Autodesk Fusion 360 part; units mm, degrees
(part 2 of 2)
sketch "Sketch5" plane through (0, 0, 14.5) normal (0, 0, 1) x (-1, 0, 0)
  line L0 (7.35, 0.35) -> (-89.35, 0.35)
  line L1 (-89.35, 0.35) -> (-89.35, -86.85)
  line L2 (-89.35, -86.85) -> (7.35, -86.85)
  line L3 (7.35, -86.85) -> (7.35, 0.35)
  spline S0 degree 3 poles (-37.3382, -76.3676) (-37.0226, -76.1422) (-36.3689, -75.6012) (-35.8504, -75.1052) knots 0 0 0 0 1 1 1 1
  line L4 (-35.8504, -75.1052) -> (-34.9262, -74.2261)
  line L5 (-34.9262, -74.2261) -> (-33.1455, -74.6093)
  spline S1 degree 3 poles (-33.1455, -74.6093) (-30.6659, -75.1278) (-28.1638, -74.97) (-26.4732, -74.2036) knots 0 0 0 0 1 1 1 1
  spline S2 degree 3 poles (-26.4732, -74.2036) (-23.385, -72.7835) (-21.5817, -69.6277) (-21.5592, -65.5928) knots 0 0 0 0 1 1 1 1
  spline S3 degree 3 poles (-21.5592, -65.5928) (-21.5366, -64.646) (-21.4014, -64.2177) (-20.6575, -63.1132) knots 0 0 0 0 1 1 1 1
  spline S4 degree 3 poles (-20.6575, -63.1132) (-19.7333, -61.7156) (-19.3726, -60.3406) (-19.6206, -59.1234) knots 0 0 0 0 1 1 1 1
  spline S5 degree 3 poles (-19.6206, -59.1234) (-19.7784, -58.2442) (-20.4321, -56.8918) (-20.6575, -56.8918) knots 0 0 0 0 1 1 1 1
  spline S6 degree 3 poles (-20.6575, -56.8918) (-20.7702, -56.8918) (-22.1002, -58.2217) (-23.633, -59.8672) knots 0 0 0 0 1 1 1 1
  spline S7 degree 3 poles (-23.633, -59.8672) (-25.1658, -61.4902) (-27.5101, -63.9923) (-28.84, -65.4124) knots 0 0 0 0 1 1 1 1
  spline S8 degree 3 poles (-28.84, -65.4124) (-30.1925, -66.8325) (-31.8381, -68.726) (-32.4918, -69.6277) knots 0 0 0 0 1 1 1 1
  spline S9 degree 3 poles (-32.4918, -69.6277) (-33.8442, -71.4535) (-35.3771, -72.8736) (-36.6168, -73.4823) knots 0 0 0 0 1 1 1 1
  spline S10 degree 3 poles (-36.6168, -73.4823) (-37.9693, -74.136) (-39.9755, -74.1134) (-46.1293, -73.3696) knots 0 0 0 0 1 1 1 1
  spline S11 degree 3 poles (-46.1293, -73.3696) (-49.2851, -72.9863) (-52.3958, -72.6031) (-53.0045, -72.5355) knots 0 0 0 0 1 1 1 1
  line L6 (-53.0045, -72.5355) -> (-54.1315, -72.4228)
  line L7 (-54.1315, -72.4228) -> (-55.3037, -74.181)
  spline S12 degree 3 poles (-55.3037, -74.181) (-56.3181, -75.6913) (-56.4308, -75.9618) (-56.0926, -76.0745) knots 0 0 0 0 1 1 1 1
  spline S13 degree 3 poles (-56.0926, -76.0745) (-55.5517, -76.2774) (-45.3178, -76.7282) (-41.2604, -76.7282) knots 0 0 0 0 1 1 1 1
  spline S14 degree 3 poles (-41.2604, -76.7282) (-38.5103, -76.7282) (-37.789, -76.6606) (-37.3382, -76.3676) knots 0 0 0 0 1 1 1 1
  spline S15 degree 3 poles (-62.1338, -75.3081) (-60.0825, -74.6995) (-57.9185, -73.4146) (-56.8591, -72.1974) knots 0 0 0 0 1 1 1 1
  spline S16 degree 3 poles (-56.8591, -72.1974) (-55.8221, -70.9576) (-54.5598, -68.5231) (-54.1315, -66.9002) knots 0 0 0 0 1 1 1 1
  spline S17 degree 3 poles (-54.1315, -66.9002) (-53.7483, -65.435) (-53.7033, -62.482) (-54.0414, -60.9492) knots 0 0 0 0 1 1 1 1
  spline S18 degree 3 poles (-54.0414, -60.9492) (-54.4697, -58.9881) (-54.5147, -58.2442) (-54.2893, -57.9737) knots 0 0 0 0 1 1 1 1
  spline S19 degree 3 poles (-54.2893, -57.9737) (-54.1766, -57.816) (-53.9512, -57.32) (-53.8385, -56.8918) knots 0 0 0 0 1 1 1 1
  spline S20 degree 3 poles (-53.8385, -56.8918) (-53.7033, -56.4635) (-52.5762, -53.1048) (-51.3139, -49.4531) knots 0 0 0 0 1 1 1 1
  spline S21 degree 3 poles (-51.3139, -49.4531) (-48.8794, -42.3976) (-48.5413, -41.3156) (-48.654, -41.248) knots 0 0 0 0 1 1 1 1
  spline S22 degree 3 poles (-48.654, -41.248) (-49.8937, -40.3463) (-54.0865, -38.6107) (-57.1972, -37.709) knots 0 0 0 0 1 1 1 1
  spline S23 degree 3 poles (-57.1972, -37.709) (-59.8796, -36.9426) (-63.1481, -36.2889) (-63.5313, -36.4467) knots 0 0 0 0 1 1 1 1
  spline S24 degree 3 poles (-63.5313, -36.4467) (-63.8244, -36.5594) (-64.2752, -37.7766) (-65.7404, -42.6907) knots 0 0 0 0 1 1 1 1
  spline S25 degree 3 poles (-65.7404, -42.6907) (-66.1236, -43.9981) (-66.5293, -45.3055) (-66.642, -45.621) knots 0 0 0 0 1 1 1 1
  spline S26 degree 3 poles (-66.642, -45.621) (-66.7547, -45.9366) (-67.0929, -47.1088) (-67.431, -48.2133) knots 0 0 0 0 1 1 1 1
  spline S27 degree 3 poles (-67.431, -48.2133) (-67.7691, -49.3404) (-68.2876, -51.031) (-68.6031, -52.0228) knots 0 0 0 0 1 1 1 1
  spline S28 degree 3 poles (-68.6031, -52.0228) (-68.8962, -52.9921) (-69.0991, -53.8261) (-69.054, -53.8937) knots 0 0 0 0 1 1 1 1
  spline S29 degree 3 poles (-69.054, -53.8937) (-68.9863, -53.9388) (-68.0396, -53.8712) (-66.9125, -53.7134) knots 0 0 0 0 1 1 1 1
  line L8 (-66.9125, -53.7134) -> (-64.8838, -53.4655)
  line L9 (-64.8838, -53.4655) -> (-63.058, -47.8526)
  spline S30 degree 3 poles (-63.058, -47.8526) (-62.0436, -44.787) (-61.1419, -42.2173) (-61.0518, -42.1497) knots 0 0 0 0 1 1 1 1
  spline S31 degree 3 poles (-61.0518, -42.1497) (-60.8263, -42.0144) (-54.943, -43.9304) (-54.65, -44.2235) knots 0 0 0 0 1 1 1 1
  spline S32 degree 3 poles (-54.65, -44.2235) (-54.4922, -44.3813) (-55.1684, -46.7256) (-56.4758, -50.6478) knots 0 0 0 0 1 1 1 1
  line L10 (-56.4758, -50.6478) -> (-58.5271, -56.8467)
  line L11 (-58.5271, -56.8467) -> (-57.9636, -57.816)
  spline S33 degree 3 poles (-57.9636, -57.816) (-56.5886, -60.2279) (-56.1152, -63.6317) (-56.8365, -66.0436) knots 0 0 0 0 1 1 1 1
  spline S34 degree 3 poles (-56.8365, -66.0436) (-57.6255, -68.7035) (-60.4206, -71.3634) (-63.3059, -72.2425) knots 0 0 0 0 1 1 1 1
  spline S35 degree 3 poles (-63.3059, -72.2425) (-64.9965, -72.7609) (-67.4535, -72.7609) (-69.1667, -72.2425) knots 0 0 0 0 1 1 1 1
  spline S36 degree 3 poles (-69.1667, -72.2425) (-71.4208, -71.5437) (-73.8328, -69.1994) (-74.8246, -66.7424) knots 0 0 0 0 1 1 1 1
  spline S37 degree 3 poles (-74.8246, -66.7424) (-75.4332, -65.2546) (-75.4783, -61.8058) (-74.8922, -60.2955) knots 0 0 0 0 1 1 1 1
  spline S38 degree 3 poles (-74.8922, -60.2955) (-74.3287, -58.7852) (-74.4188, -58.3795) (-75.3205, -57.9512) knots 0 0 0 0 1 1 1 1
  spline S39 degree 3 poles (-75.3205, -57.9512) (-75.7713, -57.7483) (-76.1545, -57.568) (-76.1996, -57.568) knots 0 0 0 0 1 1 1 1
  spline S40 degree 3 poles (-76.1996, -57.568) (-76.2447, -57.568) (-76.5828, -58.2442) (-76.9209, -59.1008) knots 0 0 0 0 1 1 1 1
  spline S41 degree 3 poles (-76.9209, -59.1008) (-77.5296, -60.4984) (-77.5746, -60.814) (-77.5521, -63.4288) knots 0 0 0 0 1 1 1 1
  spline S42 degree 3 poles (-77.5521, -63.4288) (-77.5296, -65.8407) (-77.4394, -66.4719) (-76.9886, -67.7117) knots 0 0 0 0 1 1 1 1
  spline S43 degree 3 poles (-76.9886, -67.7117) (-74.6893, -73.8429) (-68.2876, -77.1114) (-62.1338, -75.3081) knots 0 0 0 0 1 1 1 1
  spline S44 degree 3 poles (-38.037, -71.9494) (-36.8648, -71.6339) (-35.3996, -70.5293) (-34.6557, -69.4248) knots 0 0 0 0 1 1 1 1
  spline S45 degree 3 poles (-34.6557, -69.4248) (-32.2213, -65.8858) (-33.957, -60.7463) (-38.1497, -59.1459) knots 0 0 0 0 1 1 1 1
  spline S46 degree 3 poles (-38.1497, -59.1459) (-39.4571, -58.65) (-39.6149, -58.65) (-45.656, -58.7852) knots 0 0 0 0 1 1 1 1
  spline S47 degree 3 poles (-45.656, -58.7852) (-49.0597, -58.8529) (-51.945, -59.0107) (-52.0577, -59.1234) knots 0 0 0 0 1 1 1 1
  spline S48 degree 3 poles (-52.0577, -59.1234) (-52.1704, -59.2361) (-52.1479, -60.025) (-51.9676, -61.0394) knots 0 0 0 0 1 1 1 1
  spline S49 degree 3 poles (-51.9676, -61.0394) (-51.6069, -63.3837) (-51.8323, -66.2014) (-52.5762, -68.5457) knots 0 0 0 0 1 1 1 1
  spline S50 degree 3 poles (-52.5762, -68.5457) (-52.9143, -69.5826) (-53.1397, -70.4617) (-53.0946, -70.5068) knots 0 0 0 0 1 1 1 1
  spline S51 degree 3 poles (-53.0946, -70.5068) (-52.9368, -70.6646) (-40.4263, -72.2199) (-39.5923, -72.1974) knots 0 0 0 0 1 1 1 1
  spline S52 degree 3 poles (-39.5923, -72.1974) (-39.164, -72.1974) (-38.4652, -72.0847) (-38.037, -71.9494) knots 0 0 0 0 1 1 1 1
  spline S53 degree 3 poles (-64.2526, -70.6646) (-62.0887, -70.1461) (-60.105, -68.5682) (-59.023, -66.4719) knots 0 0 0 0 1 1 1 1
  spline S54 degree 3 poles (-59.023, -66.4719) (-58.482, -65.48) (-58.4144, -65.0968) (-58.4144, -63.0907) knots 0 0 0 0 1 1 1 1
  spline S55 degree 3 poles (-58.4144, -63.0907) (-58.4144, -61.0619) (-58.482, -60.7238) (-59.0456, -59.6418) knots 0 0 0 0 1 1 1 1
  spline S56 degree 3 poles (-59.0456, -59.6418) (-61.0292, -55.8774) (-65.4473, -54.3897) (-69.2343, -56.2155) knots 0 0 0 0 1 1 1 1
  spline S57 degree 3 poles (-69.2343, -56.2155) (-70.5643, -56.8692) (-72.1422, -58.4922) (-72.886, -60.0025) knots 0 0 0 0 1 1 1 1
  spline S58 degree 3 poles (-72.886, -60.0025) (-73.427, -61.1296) (-73.5172, -61.5578) (-73.5172, -63.3161) knots 0 0 0 0 1 1 1 1
  spline S59 degree 3 poles (-73.5172, -63.3161) (-73.5172, -65.1194) (-73.4496, -65.5026) (-72.8409, -66.6522) knots 0 0 0 0 1 1 1 1
  spline S60 degree 3 poles (-72.8409, -66.6522) (-71.263, -69.7855) (-67.6339, -71.4535) (-64.2526, -70.6646) knots 0 0 0 0 1 1 1 1
  spline S61 degree 3 poles (-30.1249, -64.2403) (-29.4487, -63.4513) (-27.7355, -61.4902) (-26.3154, -59.9123) knots 0 0 0 0 1 1 1 1
  spline S62 degree 3 poles (-26.3154, -59.9123) (-22.9793, -56.1254) (-22.3932, -55.3364) (-22.7088, -54.9532) knots 0 0 0 0 1 1 1 1
  spline S63 degree 3 poles (-22.7088, -54.9532) (-23.0244, -54.57) (-26.5634, -53.195) (-31.0266, -51.7072) knots 0 0 0 0 1 1 1 1
  spline S64 degree 3 poles (-31.0266, -51.7072) (-35.2869, -50.2871) (-37.0677, -50.0617) (-38.5103, -50.783) knots 0 0 0 0 1 1 1 1
  spline S65 degree 3 poles (-38.5103, -50.783) (-40.494, -51.7298) (-42.2297, -53.9839) (-42.6129, -56.0803) knots 0 0 0 0 1 1 1 1
  line L12 (-42.6129, -56.0803) -> (-42.7707, -56.9594)
  line L13 (-42.7707, -56.9594) -> (-41.4858, -56.8241)
  spline S66 degree 3 poles (-41.4858, -56.8241) (-38.8935, -56.5536) (-36.3463, -57.4778) (-34.3852, -59.3939) knots 0 0 0 0 1 1 1 1
  spline S67 degree 3 poles (-34.3852, -59.3939) (-33.1004, -60.6562) (-31.9733, -62.8652) (-31.7704, -64.5784) knots 0 0 0 0 1 1 1 1
  spline S68 degree 3 poles (-31.7704, -64.5784) (-31.7028, -65.187) (-31.5676, -65.6829) (-31.4999, -65.6604) knots 0 0 0 0 1 1 1 1
  spline S69 degree 3 poles (-31.4999, -65.6604) (-31.4323, -65.6604) (-30.8011, -65.0067) (-30.1249, -64.2403) knots 0 0 0 0 1 1 1 1
  spline S70 degree 3 poles (-59.812, -55.1561) (-59.4739, -54.5925) (-56.7013, -45.7563) (-56.7689, -45.4632) knots 0 0 0 0 1 1 1 1
  spline S71 degree 3 poles (-56.7689, -45.4632) (-56.8365, -45.1026) (-59.7669, -44.0882) (-60.0149, -44.3362) knots 0 0 0 0 1 1 1 1
  spline S72 degree 3 poles (-60.0149, -44.3362) (-60.1501, -44.4714) (-62.5846, -52.113) (-62.9002, -53.3528) knots 0 0 0 0 1 1 1 1
  spline S73 degree 3 poles (-62.9002, -53.3528) (-63.0129, -53.8712) (-62.9678, -54.0065) (-62.4719, -54.1868) knots 0 0 0 0 1 1 1 1
  spline S74 degree 3 poles (-62.4719, -54.1868) (-62.1788, -54.2995) (-61.48, -54.6151) (-60.9616, -54.863) knots 0 0 0 0 1 1 1 1
  spline S75 degree 3 poles (-60.9616, -54.863) (-59.8796, -55.3815) (-59.9472, -55.3589) (-59.812, -55.1561) knots 0 0 0 0 1 1 1 1
  spline S76 degree 3 poles (-21.1534, -52.9921) (-21.0182, -52.8343) (-19.4403, -49.7461) (-17.6369, -46.1395) knots 0 0 0 0 1 1 1 1
  line L14 (-17.6369, -46.1395) -> (-14.3459, -39.5349)
  line L15 (-14.3459, -39.5349) -> (-12.8131, -38.8135)
  spline S77 degree 3 poles (-12.8131, -38.8135) (-10.6942, -37.7766) (-8.395, -35.4549) (-7.2904, -33.2232) knots 0 0 0 0 1 1 1 1
  spline S78 degree 3 poles (-7.2904, -33.2232) (-5.8478, -30.2929) (-5.6674, -26.9567) (-6.7945, -23.7108) knots 0 0 0 0 1 1 1 1
  spline S79 degree 3 poles (-6.7945, -23.7108) (-7.9667, -20.3521) (-10.852, -17.5795) (-14.4811, -16.2946) knots 0 0 0 0 1 1 1 1
  spline S80 degree 3 poles (-14.4811, -16.2946) (-16.1943, -15.7085) (-19.6882, -15.4831) (-21.3563, -15.8663) knots 0 0 0 0 1 1 1 1
  spline S81 degree 3 poles (-21.3563, -15.8663) (-23.6555, -16.3848) (-25.8195, -17.602) (-27.5552, -19.3377) knots 0 0 0 0 1 1 1 1
  spline S82 degree 3 poles (-27.5552, -19.3377) (-30.1024, -21.8849) (-31.0266, -24.1616) (-31.3647, -28.8277) knots 0 0 0 0 1 1 1 1
  spline S83 degree 3 poles (-31.3647, -28.8277) (-31.4774, -30.5634) (-31.9733, -34.711) (-32.4918, -38.4078) knots 0 0 0 0 1 1 1 1
  spline S84 degree 3 poles (-32.4918, -38.4078) (-32.5594, -38.9713) (-32.7623, -40.4365) (-32.92, -41.6763) knots 0 0 0 0 1 1 1 1
  spline S85 degree 3 poles (-32.92, -41.6763) (-33.1004, -42.9161) (-33.3709, -44.8997) (-33.5287, -46.0944) knots 0 0 0 0 1 1 1 1
  spline S86 degree 3 poles (-33.5287, -46.0944) (-33.6865, -47.2666) (-33.7541, -48.3936) (-33.6865, -48.5965) knots 0 0 0 0 1 1 1 1
  spline S87 degree 3 poles (-33.6865, -48.5965) (-33.5963, -48.7994) (-32.5368, -49.2728) (-31.1393, -49.7461) knots 0 0 0 0 1 1 1 1
  line L16 (-31.1393, -49.7461) -> (-28.7499, -50.5576)
  line L17 (-28.7499, -50.5576) -> (-28.4343, -49.8363)
  spline S88 degree 3 poles (-28.4343, -49.8363) (-27.9384, -48.7318) (-25.256, -42.4427) (-24.1063, -39.6476) knots 0 0 0 0 1 1 1 1
  line L18 (-24.1063, -39.6476) -> (-23.0694, -37.1905)
  line L19 (-23.0694, -37.1905) -> (-23.6104, -36.8299)
  spline S89 degree 3 poles (-23.6104, -36.8299) (-27.8031, -34.0798) (-29.5388, -30.4732) (-28.795, -26.1227) knots 0 0 0 0 1 1 1 1
  spline S90 degree 3 poles (-28.795, -26.1227) (-28.0962, -22.1103) (-24.8727, -18.7742) (-20.928, -17.9176) knots 0 0 0 0 1 1 1 1
  spline S91 degree 3 poles (-20.928, -17.9176) (-15.0221, -16.6778) (-9.1614, -20.6451) (-8.2597, -26.5284) knots 0 0 0 0 1 1 1 1
  spline S92 degree 3 poles (-8.2597, -26.5284) (-7.5158, -31.3974) (-10.604, -36.1762) (-15.473, -37.5963) knots 0 0 0 0 1 1 1 1
  spline S93 degree 3 poles (-15.473, -37.5963) (-16.3295, -37.8668) (-17.4115, -37.957) (-18.9669, -37.9344) knots 0 0 0 0 1 1 1 1
  line L20 (-18.9669, -37.9344) -> (-21.221, -37.8668)
  line L21 (-21.221, -37.8668) -> (-21.9424, -39.332)
  spline S94 degree 3 poles (-21.9424, -39.332) (-22.7989, -41.0451) (-26.9691, -50.6929) (-26.9691, -50.9859) knots 0 0 0 0 1 1 1 1
  spline S95 degree 3 poles (-26.9691, -50.9859) (-26.9691, -51.0761) (-26.2252, -51.4367) (-25.3461, -51.7523) knots 0 0 0 0 1 1 1 1
  spline S96 degree 3 poles (-25.3461, -51.7523) (-24.4445, -52.0679) (-23.1821, -52.5413) (-22.5284, -52.7892) knots 0 0 0 0 1 1 1 1
  spline S97 degree 3 poles (-22.5284, -52.7892) (-21.6493, -53.1499) (-21.3112, -53.195) (-21.1534, -52.9921) knots 0 0 0 0 1 1 1 1
  spline S98 degree 3 poles (-48.0454, -38.5881) (-47.6171, -37.4385) (-47.2564, -35.9282) (-47.2564, -35.2971) knots 0 0 0 0 1 1 1 1
  spline S99 degree 3 poles (-47.2564, -35.2971) (-47.2564, -34.0573) (-48.2482, -32.3892) (-49.3528, -31.8482) knots 0 0 0 0 1 1 1 1
  spline S100 degree 3 poles (-49.3528, -31.8482) (-49.8712, -31.5777) (-50.322, -31.3298) (-50.3671, -31.3072) knots 0 0 0 0 1 1 1 1
  spline S101 degree 3 poles (-50.3671, -31.3072) (-50.3897, -31.2847) (-50.2319, -30.7211) (-49.9614, -30.09) knots 0 0 0 0 1 1 1 1
  spline S102 degree 3 poles (-49.9614, -30.09) (-49.2175, -28.1965) (-49.2626, -28.1514) (-51.3815, -27.4977) knots 0 0 0 0 1 1 1 1
  spline S103 degree 3 poles (-51.3815, -27.4977) (-54.3119, -26.5961) (-54.2668, -26.5961) (-54.8529, -28.0387) knots 0 0 0 0 1 1 1 1
  line L22 (-54.8529, -28.0387) -> (-55.3488, -29.2785)
  line L23 (-55.3488, -29.2785) -> (-56.5886, -29.2109)
  spline S104 degree 3 poles (-56.5886, -29.2109) (-58.2566, -29.1207) (-59.564, -29.7068) (-60.6686, -31.0367) knots 0 0 0 0 1 1 1 1
  spline S105 degree 3 poles (-60.6686, -31.0367) (-61.3899, -31.8933) (-62.3592, -33.8093) (-62.3592, -34.3729) knots 0 0 0 0 1 1 1 1
  spline S106 degree 3 poles (-62.3592, -34.3729) (-62.3592, -34.463) (-61.6829, -34.6434) (-60.8489, -34.8011) knots 0 0 0 0 1 1 1 1
  spline S107 degree 3 poles (-60.8489, -34.8011) (-58.8878, -35.1393) (-53.3426, -36.8524) (-50.6151, -37.9795) knots 0 0 0 0 1 1 1 1
  spline S108 degree 3 poles (-50.6151, -37.9795) (-48.2031, -38.9713) (-48.1806, -38.9713) (-48.0454, -38.5881) knots 0 0 0 0 1 1 1 1
  spline S109 degree 3 poles (-16.1492, -35.8155) (-12.4073, -34.7786) (-9.7474, -30.9015) (-10.1757, -27.092) knots 0 0 0 0 1 1 1 1
  spline S110 degree 3 poles (-10.1757, -27.092) (-10.3786, -25.3112) (-11.5958, -22.8993) (-12.8356, -21.8173) knots 0 0 0 0 1 1 1 1
  spline S111 degree 3 poles (-12.8356, -21.8173) (-15.3603, -19.6082) (-19.2825, -18.9996) (-22.2805, -20.3295) knots 0 0 0 0 1 1 1 1
  spline S112 degree 3 poles (-22.2805, -20.3295) (-27.3748, -22.5611) (-28.5695, -29.6166) (-24.5572, -33.629) knots 0 0 0 0 1 1 1 1
  spline S113 degree 3 poles (-24.5572, -33.629) (-22.3707, -35.8155) (-19.1698, -36.6495) (-16.1492, -35.8155) knots 0 0 0 0 1 1 1 1
  spline S114 degree 3 poles (-33.4385, -25.4014) (-33.3709, -25.2887) (-33.2582, -24.8604) (-33.168, -24.4321) knots 0 0 0 0 1 1 1 1
  spline S115 degree 3 poles (-33.168, -24.4321) (-32.875, -22.9894) (-31.2971, -20.0365) (-30.0798, -18.6615) knots 0 0 0 0 1 1 1 1
  spline S116 degree 3 poles (-30.0798, -18.6615) (-24.8051, -12.6655) (-16.3746, -11.6962) (-9.6122, -16.2946) knots 0 0 0 0 1 1 1 1
  line L24 (-9.6122, -16.2946) -> (-8.3273, -17.1737)
  line L25 (-8.3273, -17.1737) -> (-8.1695, -16.0241)
  spline S117 degree 3 poles (-8.1695, -16.0241) (-8.1019, -15.3704) (-8.0343, -13.5671) (-8.0343, -11.9892) knots 0 0 0 0 1 1 1 1
  line L26 (-8.0343, -11.9892) -> (-8.0343, -9.1039)
  line L27 (-8.0343, -9.1039) -> (-22.3481, -9.1039)
  line L28 (-22.3481, -9.1039) -> (-36.6619, -9.1039)
  line L29 (-36.6619, -9.1039) -> (-36.6619, -17.3315)
  line L30 (-36.6619, -17.3315) -> (-36.6619, -25.5592)
  line L31 (-36.6619, -25.5592) -> (-35.1066, -25.5592)
  spline S118 degree 3 poles (-35.1066, -25.5592) (-34.2274, -25.5592) (-33.4836, -25.4915) (-33.4385, -25.4014) knots 0 0 0 0 1 1 1 1
  line L32 (-40.1893, -6.8228) -> (-89.35, -6.8228) construction
  line L33 (-89.35, -6.8228) -> (-89.35, -25.5592) construction
  line L34 (-89.35, -25.5592) -> (-40.1893, -25.5592) construction
  line L35 (-40.1893, -25.5592) -> (-40.1893, -6.8228) construction
  dimension "d134" = 5
  text T0 "J&M AUTOMATION" font "Arial" height 5 align centre middle in box 49.1607 x 18.7363 at (-40.1893, -6.8228) x (-1, 0) y (0, -1) spacing 1
  constraint coincident L1
extrude "Extrude4'" cut sketch "Sketch5" sketch "Sketch5" against normal blind 0.2 contours S0 L4 L5 S1 S2 S3 S4 S5 S6 S7 S8 S9 S10 S11 L6 L7 S12 S13 S14 | S15 S16 S17 S18 S19 S20 S21 S22 S23 S24 S25 S26 S27 S28 S29 L8 L9 S30 S31 S32 L10 L11 S33 S34 S35 S36 S37 S38 S39 S40 S41 S42 S43 | S44 S45 S46 S47 S48 S49 S50 S51 S52 | S53 S54 S55 S56 S57 S58 S59 S60 | S61 S62 S63 S64 S65 L12 L13 S66 S67 S68 S69 | S70 S71 S72 S73 S74 S75 | S76 L14 L15 S77 S78 S79 S80 S81 S82 S83 S84 S85 S86 S87 L16 L17 S88 L18 L19 S89 S90 S91 S92 S93 L20 L21 S94 S95 S96 S97 | S98 S99 S100 S101 S102 S103 L22 L23 S104 S105 S106 S107 S108 | S109 S110 S111 S112 S113 | S114 S115 S116 L24 L25 S117 L26 L27 L28 L29 L30 L31 S118 sketch seen with x (1, 0, 0) y (0, 1, 0) z (0, 0, 1) at (0, 0, 1) of sketch 2 text T0 sketch seen with x (1, 0, 0) y (0, 1, 0) z (0, 0, 1) at (0, 0, 1) bodies 8 in component "kansi"
sketch "Sketch7" plane through (0, 0, 2) normal (0, 0, 1) x (-1, 0, 0)
  circle A0 centre (4.85, -56.85) radius 1.5
  circle A1 centre (-86.85, -56.85) radius 1.5
  circle A2 centre (4.85, -29.65) radius 1.5
  circle A3 centre (-86.85, -29.65) radius 1.5
  line L0 (-47.8333, -32.9988) -> (-47.8333, -31.9988)
  arc A4 (-47.8333, -31.9988) -> (-42.9833, -27.1469) centre (-47.8333, -27.1488) ccw
  line L1 (-42.9833, -27.1469) -> (-41.9833, -27.1465)
  arc A5 (-47.8333, -32.9988) -> (-41.9833, -27.1465) centre (-47.8333, -27.1488) ccw
  line L2 (-4.5, -32.9988) -> (-4.5, -31.9988)
  arc A6 (-4.5, -31.9988) -> (0.35, -27.1469) centre (-4.5, -27.1488) ccw
  line L3 (0.35, -27.1469) -> (1.35, -27.1465)
  arc A7 (-4.5, -32.9988) -> (1.35, -27.1465) centre (-4.5, -27.1488) ccw
  line L4 (2.35, -81.85) -> (-84.35, -81.85)
  line L5 (-84.35, -81.85) -> (-84.35, -79.85)
  line L6 (-84.35, -79.85) -> (2.35, -79.85)
  line L7 (2.35, -79.85) -> (2.35, -81.85)
  line L8 (-61.6835, -27.1499) -> (-60.6832, -27.1499)
  arc A8 (-60.6832, -27.1499) -> (-55.8332, -31.9997) centre (-55.8335, -27.15) ccw
  line L9 (-55.8332, -31.9997) -> (-55.8335, -33)
  arc A9 (-61.6835, -27.1499) -> (-55.8335, -33) centre (-55.8335, -27.15) ccw
  line L10 (-18.3501, -27.1499) -> (-17.3498, -27.1499)
  arc A10 (-17.3498, -27.1499) -> (-12.4999, -31.9997) centre (-12.5001, -27.15) ccw
  line L11 (-12.4999, -31.9997) -> (-12.5002, -33)
  arc A11 (-18.3501, -27.1499) -> (-12.5002, -33) centre (-12.5001, -27.15) ccw
  circle A12 centre (-101.85, -43.25) radius 2.5
  line L12 (-40.0168, -27.1499) -> (-39.0165, -27.1499)
  arc A13 (-39.0165, -27.1499) -> (-34.1666, -31.9997) centre (-34.1668, -27.15) ccw
  line L13 (-34.1666, -31.9997) -> (-34.1668, -33)
  arc A14 (-40.0168, -27.1499) -> (-34.1668, -33) centre (-34.1668, -27.15) ccw
  line L14 (-69.5, -32.9988) -> (-69.5, -31.9988)
  arc A15 (-69.5, -31.9988) -> (-64.65, -27.1469) centre (-69.5, -27.1488) ccw
  line L15 (-64.65, -27.1469) -> (-63.65, -27.1465)
  arc A16 (-69.5, -32.9988) -> (-63.65, -27.1465) centre (-69.5, -27.1488) ccw
  line L16 (-83.3501, -27.1499) -> (-82.3498, -27.1499)
  arc A17 (-82.3498, -27.1499) -> (-77.4999, -31.9997) centre (-77.5001, -27.15) ccw
  line L17 (-77.4999, -31.9997) -> (-77.5002, -33)
  arc A18 (-83.3501, -27.1499) -> (-77.5002, -33) centre (-77.5001, -27.15) ccw
  line L18 (-26.1667, -32.9988) -> (-26.1667, -31.9988)
  arc A19 (-26.1667, -31.9988) -> (-21.3167, -27.1469) centre (-26.1667, -27.1488) ccw
  line L19 (-21.3167, -27.1469) -> (-20.3167, -27.1465)
  arc A20 (-26.1667, -32.9988) -> (-20.3167, -27.1465) centre (-26.1667, -27.1488) ccw
  line L20 (27.35, -22.0462) -> (7.35, -2.0462)
  line L21 (7.35, -2.0462) -> (7.35, 0.35)
  line L22 (7.35, 0.35) -> (2.35, 0.35)
  line L23 (2.35, 0.35) -> (2.35, -9.85)
  line L24 (2.35, -9.85) -> (-84.35, -9.85)
  line L25 (-84.35, -9.85) -> (-84.35, 0.35)
  line L26 (-84.35, 0.35) -> (-89.35, 0.35)
  line L27 (-89.35, 0.35) -> (-89.35, -18.25)
  line L28 (-89.35, -18.25) -> (-109.35, -38.25)
  line L29 (-109.35, -38.25) -> (-109.35, -48.25)
  line L30 (-109.35, -48.25) -> (-89.35, -68.25)
  line L31 (-89.35, -68.25) -> (-89.35, -86.85)
  line L32 (-89.35, -86.85) -> (7.35, -86.85)
  line L33 (7.35, -86.85) -> (7.35, -52.0462)
  line L34 (7.35, -52.0462) -> (27.35, -32.0462)
  line L35 (27.35, -32.0462) -> (27.35, -22.0462)
sketch "Sketch8" plane through (0, -0.35, 0) normal (0, -1, 0) x (1, 0, 0)
  line L0 (17, 12) -> (17, 13)
  line L1 (17, 13) -> (21.6675, 13)
  line L2 (21.6675, 13) -> (21.6675, 12)
  line L3 (21.6675, 12) -> (38.6675, 12)
  line L4 (38.6675, 12) -> (38.6675, 13)
  line L5 (38.6675, 13) -> (43.335, 13)
  line L6 (43.335, 13) -> (43.335, 12)
  line L7 (43.335, 12) -> (60.335, 12)
  line L8 (60.335, 12) -> (60.335, 13)
  line L9 (60.335, 13) -> (65.0025, 13)
  line L10 (65.0025, 13) -> (65.0025, 12)
  line L11 (65.0025, 12) -> (82, 12)
  line L12 (82, 12) -> (82, 13)
  line L13 (82, 13) -> (84.35, 13)
  line L14 (84.35, 13) -> (84.35, 2)
  line L15 (84.35, 2) -> (89.35, 2)
  line L16 (89.35, 2) -> (89.35, 14.5)
  line L17 (89.35, 14.5) -> (-7.35, 14.5)
  line L18 (-7.35, 14.5) -> (-7.35, 2)
  line L19 (-7.35, 2) -> (-2.35, 2)
  line L20 (-2.35, 2) -> (-2.35, 13)
  line L21 (-2.35, 13) -> (0, 13)
  line L22 (0, 13) -> (0, 12)
  line L23 (0, 12) -> (17, 12)
  circle A0 centre (-10.1, 10.25) radius 2.75
  line L24 (-7.35, 13) -> (-7.35, 14.5)
  line L25 (-7.35, 7.6) -> (-7.35, 6)
  line L26 (-7.35, 14.5) -> (-13.35, 14.5)
  line L27 (-7.35, 6) -> (-13.35, 6)
  line L28 (-13.35, 14.5) -> (-13.35, 12.5)
  line L29 (-13.35, 6) -> (-13.35, 8)
  line L30 (-13.35, 8) -> (-11.6811, 8)
  line L31 (-13.35, 12.5) -> (-11.6811, 12.5)
  point P0 (-4.85, 2)
  dimension "d135" = 5.5
  dimension "d136" = 2.75
  dimension "d140" = 6
  dimension "d141" = 6
  dimension "d142" = 2
  dimension "d143" = 2
  dimension "d146" = 4.25
  dimension "d154" = 4.25
  constraint coincident L18 L24.start
  constraint coincident L18 L25.start
  constraint perpendicular L19 L25
  constraint perpendicular L18 L26
  constraint perpendicular L18 L27
  constraint perpendicular L26 L28
  constraint perpendicular L27 L29
  constraint coincident A0 L30.end
  constraint perpendicular L29 L30
  constraint coincident A0 L31.end
  constraint perpendicular L28 L31
  constraint coincident L17.end L18.start
  measures "d135" diameter of A0
  measures "d136" distance of L18 A0.centre
  measures "d140" distance of L17.end L26.end
  measures "d141" distance of L25.end L27.end
  measures "d142" distance of L26.end L28.end
  measures "d143" distance of L27.end L29.end
  measures "d146" distance of L17 A0.centre
  measures "d154" distance of A0.centre L27
extrude "Extrude6'" add sketch "Sketch8" against normal blind 15 contours L18 A0 L25 L27 L29 L30 | L18 A0 L24 L26 L28 L31 sketch seen with x (1, 0, 0) y (0, 1, 0) z (0, 0, 1) at (0, 0, 1) bodies 8 in component "kansi"
sketch "Sketch9" plane through (0, 86.85, 0) normal (0, 1, 0) x (-1, 0, 0)
  line L0 (-89.35, 14.5) -> (-89.35, 2)
  line L1 (-89.35, 2) -> (7.35, 2)
  line L2 (7.35, 2) -> (7.35, 14.5)
  line L3 (7.35, 14.5) -> (-89.35, 14.5)
  line L4 (-49, 2) -> (-33, 2)
  line L5 (-33, 2) -> (-33, 6)
  line L6 (-33, 6) -> (-49, 6)
  line L7 (-49, 6) -> (-49, 2)
  dimension "d147" = 16
  dimension "d148" = 4
  dimension "d149" = 40.35
  constraint horizontal L4
  constraint vertical L5
  constraint horizontal L6
  constraint vertical L7
  constraint coincident L1 L4.start
  measures "d147" distance of L4.start L4.end
  measures "d148" distance of L4.start L6.end
  measures "d149" distance of L0 L7
extrude "Extrude3''" cut sketch "Sketch9" against normal blind 10 contours L1 L4 L5 L6 L7 bodies 7 in component "boksi"
extrude "Extrude7'" cut sketch "Sketch9" against normal blind 10 contours L1 L4 L5 L6 L7 sketch seen with x (1, 0, 0) y (0, 1, 0) z (0, 0, 1) at (0, 0, 1) bodies 8 in component "kansi"
component "boksi" placed x (1, 0, 0) y (0, 1, 0) z (0, 0, 1) at (0, 0, 0)
component "kansi" placed x (1, 0, 0) y (0, 1, 0) z (0, 0, 1) at (0, 0, -1)
equation "d56 = 9 mm + ( 0.35 * 2 ) * 1 mm + 0.5 mm"
equation "d95 = ( 35.3799163327 mm + 41.82 mm ) / 2"
equation "d107 = 1 mm + 1.5 mm"
equation "d110 = 1 mm + 1.5 mm"
equation "d114 = 1 mm + 1.5 mm"
equation "d117 = 1 mm + 1.5 mm"
equation "d118 = 5 mm - 0.6 mm"
equation "d119 = 5 mm - 0.6 mm"
equation "d120 = 5 mm - 0.6 mm"
equation "d121 = 5 mm - 0.6 mm"
equation "d122 = -2 mm - 6 mm"
equation "d124 = -2 mm - 6 mm"
equation "d136 = ( 5.5 / 2 ) * 1 mm"
equation "d141 = 5.5 mm + 0.5 mm"
equation "d146 = ( 5.5 / 2 ) * 1 mm + 1.5 mm"
equation "d147 = ( 4 * 4 ) * 1 mm"
equation "d149 = ( 30 mm + 50.70 mm ) / 2"
equation "d154 = ( 5.5 / 2 ) * 1 mm + 1.5 mm"
